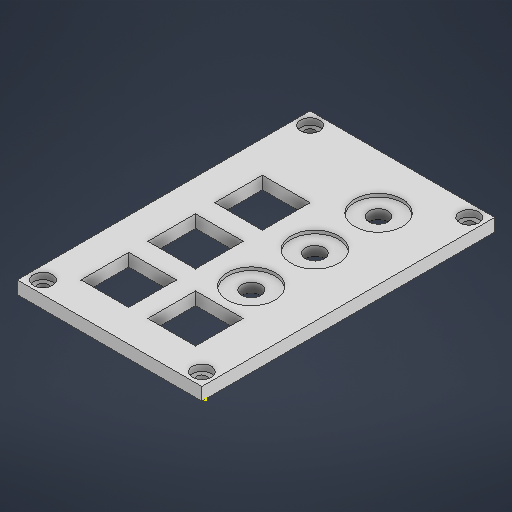
# Autodesk Inventor part: streamdeck lid
Saved by Autodesk Inventor 2026.1 (Build 301233020, 233B)
## iProperties
Created: 2026-08-22
Part Number: streamdeck lid
Material: Generic
Document SubType Name: Modeling
Designer: joppo
Density: 1 g/cm^3
Appearance: Default
Author: joppo
Autodesk Inventor part; units mm, degrees
ref_plane "YZ Plane" through (0, 0, 0) normal (1, 0, 0) x (0, 1, 0)
ref_plane "XZ Plane" through (0, 0, 0) normal (0, 1, 0) x (-1, 0, 0)
ref_plane "XY Plane" through (0, 0, 0) normal (0, 0, 1) x (1, 0, 0)
sketch "Sketch1" plane through (0, 0, 0) normal (0, 1, 0) x (-1, 0, 0)
  line L0 (0, 0) -> (0, -90)
  line L1 (0, -90) -> (56, -90)
  line L2 (56, -90) -> (56, 0)
  line L3 (56, 0) -> (0, 0)
  dimension "d0" = 90
  dimension "d1" = 56
  constraints: 8 end point, 2 perpendicular, 1 horizontal, 1 vertical
  measures "d0" distance of L0.start L0.end
  measures "d1" distance of L0.end L1.end
extrude "Extrusion1" add sketch "Sketch1" along normal blind 4
sketch "Sketch2" plane through (0, 4, 0) normal (0, 1, 0) x (1, 0, 0)
  circle A0 centre (-3, 3) radius 3
  circle A1 centre (-52.9351, 2.9993) radius 3
  circle A2 centre (-53, 87) radius 3
  circle A3 centre (-3, 87) radius 3
  point P0 (0, 0)
  point P1 (-56, 0)
  point P2 (0, 90)
  point P3 (-56, 90)
  dimension "d6" = 6
  dimension "d17" = 6
  dimension "d20" = 6
  dimension "d23" = 6
  constraints: 4 centre point
  measures "d6" diameter of A0
  measures "d17" diameter of A1
  measures "d20" diameter of A2
  measures "d23" diameter of A3
sketch "Sketch5" plane through (0, 0, -90) normal (0, 0, -1) x (-1, 0, 0)
  line L0 (0, 0) -> (56, 0) projected
  line L1 (0, 0) -> (56, 0)
  line L2 (56, 0) -> (56, 4) projected
  line L3 (56, 0) -> (56, 4)
  line L4 (56, 4) -> (0, 4)
  line L5 (0, 0) -> (0, 4) projected
  line L6 (0, 0) -> (0, 4)
  constraints: 8 end point, 2 perpendicular, 1 collinear, 1 horizontal
extrude "Extrusion2" add sketch "Sketch5" along normal blind 1
sketch "Sketch7" plane through (-56, 0, 0) normal (0, 0, 1) x (1, 0, 0)
  line L0 (0, 0) -> (0, 4) projected
  line L1 (0, 4) -> (0, 0)
  line L2 (0, 0) -> (56, 0)
  line L3 (56, 0) -> (56, 4)
  line L4 (56, 4) -> (0, 4)
  constraints: 8 end point, 3 perpendicular, 1 collinear
extrude "Extrusion3" add sketch "Sketch7" along normal blind 1
sketch "Sketch8" plane through (0, 0, -91) normal (1, 0, 0) x (0, 0, -1)
  line L0 (-92, 0) -> (-92, 4) projected
  line L1 (0, 0) -> (-92, 0) projected
  line L2 (-92, 4) -> (-92, 0)
  line L3 (-92, 0) -> (0, 0)
  line L4 (0, 4) -> (0, 0) projected
  line L5 (0, 0) -> (0, 4)
  line L6 (0, 4) -> (-92, 4) projected
  line L7 (0, 4) -> (-92, 4)
  point P0 (-91, 0)
  constraints: 8 end point, 3 perpendicular, 1 collinear
extrude "Extrusion4" add sketch "Sketch8" along normal blind 1
sketch "Sketch9" plane through (-56, 0, -91) normal (-1, 0, 0) x (0, 0, 1)
  line L0 (92, 0) -> (0, 0) projected
  line L1 (92, 4) -> (92, 0) projected
  line L2 (0, 0) -> (92, 0)
  line L3 (92, 0) -> (92, 4)
  line L4 (92, 4) -> (0, 4)
  line L5 (0, 4) -> (0, 0)
  point P0 (91, 0)
  constraints: 8 end point, 3 perpendicular, 1 horizontal
extrude "Extrusion5" add sketch "Sketch9" along normal blind 1
sketch "Sketch10" plane through (1, 0, -91) normal (1, 0, 0) x (0, 0, -1)
  point P0 (-91, 0)
extrude "Extrusion6" cut sketch "Sketch2" against normal blind 2
sketch "Sketch11" plane through (-3, 2, -87) normal (0, 1, 0) x (1, 0, 0)
  circle A0 centre (0, -84) radius 3 projected
  circle A1 centre (0, -84) radius 1.6
  circle A2 centre (-49.9351, -84.0007) radius 3 projected
  circle A3 centre (-49.9351, -84.0007) radius 1.6
  circle A4 centre (-50, 0) radius 3 projected
  circle A5 centre (-50, 0) radius 1.6
  circle A6 centre (0, 0) radius 3 projected
  circle A7 centre (0, 0) radius 1.6
  point P0 (3, -87)
  dimension "d26" = 3.2
  dimension "d27" = 3.2
  dimension "d28" = 3.2
  dimension "d29" = 3.2
  constraints: 4 centre point, 4 coincident
  measures "d26" diameter of A1
  measures "d27" diameter of A3
  measures "d28" diameter of A5
  measures "d29" diameter of A7
extrude "Extrusion7" cut sketch "Sketch11" against normal blind 2 contours A1 | A3 | A5 | A7
sketch "Sketch12" plane through (0, 4, 0) normal (0, 1, 0) x (1, 0, 0)
  line L0 (-47, 9) -> (-47, 24)
  line L1 (-47, 24) -> (-32, 24)
  line L2 (-32, 24) -> (-32, 9)
  line L3 (-32, 9) -> (-47, 9)
  line L4 (-47, 30) -> (-32, 30)
  line L5 (-32, 30) -> (-32, 45)
  line L6 (-32, 45) -> (-47, 45)
  line L7 (-47, 45) -> (-47, 30)
  line L8 (-47, 51) -> (-47, 66)
  line L9 (-47, 66) -> (-32, 66)
  line L10 (-32, 66) -> (-32, 51)
  line L11 (-32, 51) -> (-47, 51)
  line L12 (-57, 91) -> (1, 91) projected
  line L13 (-26, 9) -> (-26, 24)
  line L14 (-26, 24) -> (-11, 24)
  line L15 (-11, 24) -> (-11, 9)
  line L16 (-11, 9) -> (-26, 9)
  circle A0 centre (-18.5, 34) radius 3
  circle A1 centre (-18.5, 54) radius 3
  circle A2 centre (-18.5, 74) radius 3
  line L17 (-18.5, 54) -> (-18.5, 74)
  point P0 (0, 0)
  point P1 (-57, -1)
  dimension "d34" = 15
  dimension "d35" = 15
  dimension "d37" = 15
  dimension "d39" = 15
  dimension "d44" = 15
  dimension "d46" = 6
  dimension "d48" = 6
  dimension "d50" = 6
  dimension "d57" = 20
  constraints: 34 end point, 12 perpendicular, 4 vertical, 3 centre point, 1 horizontal
  measures "d34" distance of L0.start L0.end
  measures "d35" distance of L0.end L1.end
  measures "d37" distance of L4.end L5.end
  measures "d39" distance of L8.start L8.end
  measures "d44" distance of L13.end L14.end
  measures "d46" diameter of A0
  measures "d48" diameter of A1
  measures "d50" diameter of A2
  measures "d57" distance of L17.start L17.end
extrude "Extrusion8" cut sketch "Sketch12" against normal blind 4
sketch "Sketch13" plane through (0, 4, 0) normal (0, 1, 0) x (1, 0, 0)
  circle A0 centre (-18.5, 34) radius 3 projected
  circle A1 centre (-18.5, 34) radius 7.5
  circle A2 centre (-18.5, 54) radius 3 projected
  circle A3 centre (-18.5, 54) radius 7.5
  circle A4 centre (-18.5, 74) radius 3 projected
  circle A5 centre (-18.5, 74) radius 7.5
  point P0 (0, 0)
  dimension "d58" = 15
  dimension "d59" = 15
  dimension "d60" = 15
  constraints: 3 centre point, 3 coincident
  measures "d58" diameter of A1
  measures "d59" diameter of A3
  measures "d60" diameter of A5
extrude "Extrusion9" cut sketch "Sketch13" against normal blind 1
body "Solid1"
